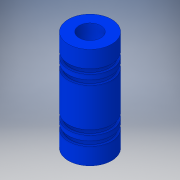
# Autodesk Inventor part: Roller-ver3-1111-2019
Saved by Autodesk Inventor 2018 (Build 220112000, 112)
## iProperties
Created: 2020-01-25
Part Number: Roller-ver3-1111-2019
Material: Generic
Document SubType Name: Modeling
Designer: JMHal
Density: 1 g/cm^3
Appearance: Default
Author: JMHal
Autodesk Inventor part; units mm, degrees
ref_plane "YZ Plane" through (0, 0, 0) normal (1, 0, 0) x (0, 1, 0)
ref_plane "XZ Plane" through (0, 0, 0) normal (0, 1, 0) x (-1, 0, 0)
ref_plane "XY Plane" through (0, 0, 0) normal (0, 0, 1) x (1, 0, 0)
sketch "Sketch1" plane through (0, 0, 0) normal (0, 1, 0) x (-1, 0, 0)
  circle A0 centre (0, 0) radius 28.575
  circle A1 centre (0, 0) radius 14.2875
  dimension "d0" = 57.15
  dimension "d1" = 28.575
  constraints: 2 centre point, 2 coincident
  measures "d0" diameter of A0
  measures "d1" diameter of A1
extrude "Extrusion1" add sketch "Sketch1" along normal blind 50.8
sketch "Sketch2" plane through (0, 0, 0) normal (0, -1, 0) x (1, 0, 0)
  circle A0 centre (0, 0) radius 22.225
  circle A1 centre (0, 0) radius 14.2875
  dimension "d6" = 28.575
  constraints: 2 centre point, 2 coincident
  measures "d6" diameter of A1
extrude "Extrusion2" add sketch "Sketch2" along normal blind 6.35
sketch "Sketch3" plane through (0, -6.35, 0) normal (0, -1, 0) x (1, 0, 0)
  circle A0 centre (0, 0) radius 28.575
  circle A1 centre (0, 0) radius 14.2875
  dimension "d9" = 57.15
  dimension "d10" = 28.575
  constraints: 2 centre point, 2 coincident
  measures "d9" diameter of A0
  measures "d10" diameter of A1
extrude "Extrusion3" add sketch "Sketch3" along normal blind 6.35
sketch "Sketch4" plane through (0, 50.8, 0) normal (0, 1, 0) x (1, 0, 0)
  circle A0 centre (0, 0) radius 22.225
  circle A1 centre (0, 0) radius 14.2875
  dimension "d15" = 28.575
  constraints: 2 centre point, 2 coincident
  measures "d15" diameter of A1
extrude "Extrusion4" add sketch "Sketch4" along normal blind 6.35
sketch "Sketch5" plane through (0, 57.15, 0) normal (0, 1, 0) x (1, 0, 0)
  circle A0 centre (0, 0) radius 28.575
  circle A1 centre (0, 0) radius 14.2875
  dimension "d18" = 57.15
  dimension "d19" = 28.575
  constraints: 2 centre point, 2 coincident
  measures "d18" diameter of A0
  measures "d19" diameter of A1
extrude "Extrusion5" add sketch "Sketch5" along normal blind 6.35
sketch "Sketch6" plane through (0, -12.7, 0) normal (0, -1, 0) x (1, 0, 0)
  circle A0 centre (0, 0) radius 22.225
  circle A1 centre (0, 0) radius 14.2875
  dimension "d24" = 28.575
  constraints: 2 centre point, 2 coincident
  measures "d24" diameter of A1
extrude "Extrusion6" add sketch "Sketch6" along normal blind 6.35
sketch "Sketch7" plane through (0, 63.5, 0) normal (0, 1, 0) x (1, 0, 0)
  circle A0 centre (0, 0) radius 22.225
  circle A1 centre (0, 0) radius 14.2875
  dimension "d29" = 28.575
  constraints: 2 centre point, 2 coincident
  measures "d29" diameter of A1
extrude "Extrusion7" add sketch "Sketch7" along normal blind 6.35
sketch "Sketch8" plane through (0, 69.85, 0) normal (0, 1, 0) x (1, 0, 0)
  circle A0 centre (0, 0) radius 28.575
  circle A1 centre (0, 0) radius 14.2875
  dimension "d32" = 57.15
  dimension "d33" = 28.575
  constraints: 2 centre point, 2 coincident
  measures "d32" diameter of A0
  measures "d33" diameter of A1
extrude "Extrusion8" add sketch "Sketch8" along normal blind 22.225
sketch "Sketch9" plane through (0, -19.05, 0) normal (0, -1, 0) x (1, 0, 0)
  circle A0 centre (0, 0) radius 28.575
  circle A1 centre (0, 0) radius 28.575 projected
  circle A2 centre (0, 0) radius 14.2875
  dimension "d36" = 57.15
  dimension "d37" = 28.575
  constraints: 2 centre point, 2 coincident
  measures "d36" diameter of A0
  measures "d37" diameter of A2
extrude "Extrusion9" add sketch "Sketch9" along normal blind 22.225
fillet "Fillet2" radius 3.175 8 edges at (-22.225, -19.05, 0) (-22.225, -12.7, 0) (-22.225, 0, 0) (-22.225, -6.35, 0) (-22.225, 50.8, 0) (-22.225, 57.15, 0) (-22.225, 69.85, 0) (-22.225, 63.5, 0)
body "Solid1"
